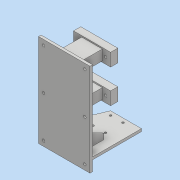
# Autodesk Inventor part: Giá đỡ động cơ
Saved by Autodesk Inventor 2018 (Build 220112000, 112)
## iProperties
Created: 2020-08-22
Part Number: Giá đỡ động cơ
Material: Generic
Document SubType Name: Modeling
Designer: ASUS
Density: 1 g/cm^3
Appearance: Default
Author: ASUS
Autodesk Inventor part; units mm, degrees
ref_plane "YZ Plane" through (0, 0, 0) normal (1, 0, 0) x (0, 1, 0)
ref_plane "XZ Plane" through (0, 0, 0) normal (0, 1, 0) x (-1, 0, 0)
ref_plane "XY Plane" through (0, 0, 0) normal (0, 0, 1) x (1, 0, 0)
sketch "Sketch1" plane through (0, 0, 0) normal (0, 1, 0) x (-1, 0, 0)
  line L0 (0, 0) -> (100, 0)
  line L1 (100, 0) -> (100, -180)
  line L2 (100, -180) -> (0, -180)
  line L3 (0, -180) -> (0, 0)
  dimension "d0" = 100
  dimension "d1" = 180
  constraints: 8 end point, 2 parallel, 1 horizontal, 1 perpendicular
  measures "d0" distance of L1.end L2.end
  measures "d1" distance of L0.end L1.end
extrude "Extrusion1" add sketch "Sketch1" along normal blind 5
sketch "Sketch2" plane through (0, 5, 0) normal (0, 1, 0) x (1, 0, 0)
  line L0 (0, 160) -> (-100, 160)
  line L1 (-100, 160) -> (-100, 155)
  line L2 (-100, 155) -> (0, 155)
  line L3 (0, 155) -> (0, 160)
  line L4 (0, 180) -> (-100, 180) projected
  point P0 (0, 0)
  dimension "d4" = 100
  dimension "d5" = 5
  dimension "d6" = 20
  constraints: 8 end point, 2 parallel, 1 horizontal, 1 perpendicular
  measures "d4" distance of L2.end L1.end
  measures "d5" distance of L1.end L0.end
  measures "d6" distance between parallel lines of L4 L0
extrude "Extrusion2" add sketch "Sketch2" along normal blind 95
sketch "Sketch5" plane through (0, 5, -160) normal (0, 0, -1) x (-1, 0, 0)
  line L0 (28, 87) -> (52, 87)
  line L1 (52, 87) -> (52, 53)
  line L2 (52, 53) -> (28, 53)
  line L3 (28, 53) -> (28, 87)
  line L4 (28, 87) -> (52, 53) construction
  line L5 (52, 87) -> (28, 53) construction
  line L6 (0, 0) -> (0, 95) projected
  line L7 (0, 95) -> (100, 95) projected
  circle A0 centre (28, 87) radius 2
  circle A1 centre (52, 87) radius 2
  circle A2 centre (28, 53) radius 2
  circle A3 centre (52, 53) radius 2
  point P0 (0, -5)
  point P1 (40, 70)
  point P2 (50, 95)
  dimension "d14" = 24
  dimension "d15" = 34
  dimension "d16" = 40
  dimension "d17" = 25
  dimension "d19" = 4
  dimension "d20" = 4
  dimension "d21" = 4
  dimension "d22" = 4
  constraints: 12 end point, 4 centre point, 4 coincident, 2 midpoint, 2 parallel, 1 horizontal, 1 perpendicular
  measures "d14" distance of L1.end L2.end
  measures "d15" distance of L0.end L1.end
  measures "d16" distance from line of L6 point (40, 70)
  measures "d17" distance from line of L7 point (40, 70)
  measures "d19" diameter of A0
  measures "d20" diameter of A1
  measures "d21" diameter of A2
  measures "d22" diameter of A3
extrude "Extrusion4" cut sketch "Sketch5" against normal blind 95 contours L3 A0 L0 | L0 A0 L3 | A1 L1 L0 | L0 L1 A1 | A2 L2 L3 | L3 L2 A2 | A3 L2 L1 | L1 L2 A3
sketch "Sketch12" plane through (0, 5, -160) normal (0, 0, -1) x (-1, 0, 0)
  line L0 (0, 95) -> (100, 95) projected
  line L1 (100, 95) -> (60, 95)
  line L2 (100, 0) -> (0, 0) projected
  line L3 (60, 95) -> (100, 0)
  line L4 (100, 0) -> (100, 95)
  point P0 (0, -5)
  dimension "d72" = 40
  constraints: 6 end point, 1 perpendicular, 1 point on line
  measures "d72" distance of L0.end L1.end
extrude "Extrusion10" cut sketch "Sketch12" against normal blind 14
sketch "Sketch13" plane through (0, 5, 0) normal (0, 1, 0) x (1, 0, 0)
  line L0 (-20, 23) -> (-60, 23)
  line L1 (-60, 23) -> (-60, 3)
  line L2 (-60, 3) -> (-20, 3)
  line L3 (-20, 3) -> (-20, 23)
  line L4 (-20, 23) -> (-60, 3) construction
  line L5 (-60, 23) -> (-20, 3) construction
  line L6 (-100, 0) -> (0, 0) projected
  line L7 (0, 0) -> (0, 155) projected
  line L8 (-20, 88) -> (-60, 88)
  line L9 (-60, 88) -> (-60, 68)
  line L10 (-60, 68) -> (-20, 68)
  line L11 (-20, 68) -> (-20, 88)
  line L12 (-20, 88) -> (-60, 68) construction
  line L13 (-60, 88) -> (-20, 68) construction
  point P0 (-40, 13)
  point P1 (-40, 78)
  dimension "d76" = 40
  dimension "d77" = 20
  dimension "d78" = 3
  dimension "d79" = 40
  dimension "d80" = 40
  dimension "d81" = 20
  dimension "d82" = 45
  dimension "d83" = 40
  constraints: 24 end point, 4 midpoint, 4 parallel, 2 horizontal, 2 perpendicular
  measures "d76" distance of L2.end L1.end
  measures "d77" distance of L1.end L0.end
  measures "d78" distance between parallel lines of L6 L2
  measures "d79" distance from line of L7 point (-40, 13)
  measures "d80" distance of L10.end L9.end
  measures "d81" distance of L9.end L8.end
  measures "d82" distance between parallel lines of L0 L10
  measures "d83" distance from line of L7 point (-40, 78)
extrude "Extrusion11" add sketch "Sketch13" along normal blind 39
sketch "Sketch14" plane through (0, 44, 0) normal (0, 1, 0) x (1, 0, 0)
  line L0 (-4, 90.5) -> (-76, 90.5)
  line L1 (-76, 90.5) -> (-76, 65.5)
  line L2 (-76, 65.5) -> (-4, 65.5)
  line L3 (-4, 65.5) -> (-4, 90.5)
  line L4 (-4, 90.5) -> (-76, 65.5) construction
  line L5 (-76, 90.5) -> (-4, 65.5) construction
  line L6 (-20, 88) -> (-60, 88) projected
  line L7 (-20, 68) -> (-20, 88) projected
  line L8 (-4, 25.5) -> (-76, 25.5)
  line L9 (-76, 25.5) -> (-76, 0.5)
  line L10 (-76, 0.5) -> (-4, 0.5)
  line L11 (-4, 0.5) -> (-4, 25.5)
  line L12 (-4, 25.5) -> (-76, 0.5) construction
  line L13 (-76, 25.5) -> (-4, 0.5) construction
  line L14 (-20, 23) -> (-60, 23) projected
  line L15 (-20, 3) -> (-20, 23) projected
  point P0 (0, 0)
  point P1 (-40, 78)
  point P2 (-40, 13)
  dimension "d86" = 72
  dimension "d87" = 25
  dimension "d88" = 10
  dimension "d89" = 20
  dimension "d90" = 72
  dimension "d91" = 25
  dimension "d92" = 10
  dimension "d93" = 20
  constraints: 24 end point, 4 midpoint, 4 parallel, 2 horizontal, 2 perpendicular
  measures "d86" distance of L2.end L1.end
  measures "d87" distance of L1.end L0.end
  measures "d88" distance from line of L6 point (-40, 78)
  measures "d89" distance from line of L7 point (-40, 78)
  measures "d90" distance of L10.end L9.end
  measures "d91" distance of L9.end L8.end
  measures "d92" distance from line of L14 point (-40, 13)
  measures "d93" distance from line of L15 point (-40, 13)
extrude "Extrusion12" add sketch "Sketch14" along normal blind 14
sketch "Sketch16" plane through (0, 5, 0) normal (0, 1, 0) x (1, 0, 0)
  line L0 (0, 180) -> (-100, 180) projected
  line L1 (-38, 160) -> (-43, 160)
  line L2 (-43, 160) -> (-43, 180)
  line L3 (-43, 180) -> (-38, 180)
  line L4 (-38, 180) -> (-38, 160)
  line L5 (0, 160) -> (0, 180) projected
  point P0 (0, 0)
  dimension "d96" = 20
  dimension "d97" = 38
  dimension "d98" = 5
  constraints: 8 end point, 2 parallel, 1 horizontal, 1 perpendicular, 1 point on line
  measures "d96" distance of L3.end L1.start
  measures "d97" distance between parallel lines of L5 L4
  measures "d98" distance between parallel lines of L4 L2
extrude "Extrusion13" add sketch "Sketch16" along normal blind 95
sketch "Sketch18" plane through (0, 5, 0) normal (0, 1, 0) x (1, 0, 0)
  line L0 (-60, 155) -> (-100, 155) projected
  line L1 (-82, 155) -> (-77, 155)
  line L2 (-77, 155) -> (-77, 125)
  line L3 (-77, 125) -> (-82, 125)
  line L4 (-82, 125) -> (-82, 155)
  line L5 (-23, 155) -> (-18, 155)
  line L6 (-18, 155) -> (-18, 125)
  line L7 (-18, 125) -> (-23, 125)
  line L8 (-23, 125) -> (-23, 155)
  line L9 (-100, 155) -> (-100, 0) projected
  line L10 (0, 0) -> (0, 155) projected
  dimension "d103" = 5
  dimension "d104" = 30
  dimension "d105" = 5
  dimension "d106" = 30
  dimension "d107" = 18
  dimension "d108" = 18
  constraints: 16 end point, 4 parallel, 2 horizontal, 2 perpendicular, 2 point on line
  measures "d103" distance of L2.end L3.end
  measures "d104" distance of L1.end L2.end
  measures "d105" distance of L6.end L7.end
  measures "d106" distance of L5.end L6.end
  measures "d107" distance between parallel lines of L9 L4
  measures "d108" distance between parallel lines of L10 L6
extrude "Extrusion15" add sketch "Sketch18" along normal blind 40
sketch "Sketch20" plane through (-43, 5, -180) normal (-1, 0, 0) x (0, 0, 1)
  line L0 (20, 0) -> (20, 95) projected
  line L1 (20, 95) -> (20, 65)
  line L2 (20, 65) -> (15, 65)
  line L3 (0, 0) -> (20, 0) projected
  line L4 (15, 65) -> (0, 0)
  line L5 (0, 95) -> (20, 95) projected
  line L6 (0, 0) -> (0, 95)
  line L7 (0, 95) -> (20, 95)
  point P0 (180, -5)
  dimension "d114" = 30
  dimension "d115" = 5
  constraints: 10 end point, 2 perpendicular, 1 horizontal, 1 point on line
  measures "d114" distance of L0.end L1.end
  measures "d115" distance of L1.end L2.end
extrude "Extrusion17" cut sketch "Sketch20" against normal blind 10 contours L2 L4 L6 L5 L0
sketch "Sketch21" plane through (0, 5, 0) normal (0, 1, 0) x (1, 0, 0)
  circle A0 centre (-90, 10) radius 2.5
  line L0 (-100, 155) -> (-100, 0) projected
  line L1 (-100, 0) -> (0, 0) projected
  circle A1 centre (-10, 10) radius 2.5
  line L2 (0, 0) -> (0, 155) projected
  circle A2 centre (-90, 170) radius 2.5
  line L3 (-43, 180) -> (-100, 180) projected
  line L4 (-100, 180) -> (-100, 160) projected
  circle A3 centre (-10, 170) radius 2.5
  line L5 (0, 180) -> (-38, 180) projected
  line L6 (0, 160) -> (0, 180) projected
  circle A4 centre (-50, 50) radius 2.5
  circle A5 centre (-50, 130) radius 2.5
  dimension "d118" = 5
  dimension "d119" = 10
  dimension "d120" = 10
  dimension "d121" = 5
  dimension "d122" = 10
  dimension "d123" = 10
  dimension "d124" = 5
  dimension "d125" = 10
  dimension "d126" = 10
  dimension "d127" = 5
  dimension "d128" = 10
  dimension "d129" = 10
  dimension "d130" = 5
  dimension "d131" = 5
  dimension "d132" = 50
  dimension "d133" = 50
  constraints: 6 centre point
  measures "d118" diameter of A0
  measures "d119" distance from line of L0 A0.centre
  measures "d120" distance from line of L1 A0.centre
  measures "d121" diameter of A1
  measures "d122" distance from line of L2 A1.centre
  measures "d123" distance from line of L1 A1.centre
  measures "d124" diameter of A2
  measures "d125" distance from line of L3 A2.centre
  measures "d126" distance from line of L4 A2.centre
  measures "d127" diameter of A3
  measures "d128" distance from line of L5 A3.centre
  measures "d129" distance from line of L6 A3.centre
  measures "d130" diameter of A4
  measures "d131" diameter of A5
  measures "d132" distance from line of L1 A4.centre
  measures "d133" distance from line of L3 A5.centre
extrude "Extrusion18" cut sketch "Sketch21" against normal blind 10
sketch "Sketch27" plane through (0, 58, 0) normal (0, 1, 0) x (1, 0, 0)
  circle A0 centre (-66.5, 78) radius 2.5
  line L0 (-4, 90.5) -> (-76, 90.5) projected
  line L1 (-76, 90.5) -> (-76, 65.5) projected
  circle A1 centre (-13.5, 78) radius 2.5
  line L2 (-76, 65.5) -> (-4, 65.5) projected
  circle A2 centre (-66.5, 13) radius 2.5
  line L3 (-76, 25.5) -> (-76, 0.5) projected
  line L4 (-76, 0.5) -> (-4, 0.5) projected
  circle A3 centre (-13.5, 13) radius 2.5
  line L5 (-4, 0.5) -> (-4, 25.5) projected
  point P0 (0, 0)
  dimension "d137" = 5
  dimension "d138" = 12.5
  dimension "d139" = 9.5
  dimension "d140" = 5
  dimension "d141" = 53
  dimension "d142" = 12.5
  dimension "d143" = 5
  dimension "d144" = 9.5
  dimension "d145" = 12.5
  dimension "d146" = 5
  dimension "d147" = 9.5
  dimension "d148" = 12.5
  constraints: 4 centre point
  measures "d137" diameter of A0
  measures "d138" distance from line of L0 A0.centre
  measures "d139" distance from line of L1 A0.centre
  measures "d140" diameter of A1
  measures "d141" distance of A0.centre A1.centre
  measures "d142" distance from line of L2 A1.centre
  measures "d143" diameter of A2
  measures "d144" distance from line of L3 A2.centre
  measures "d145" distance from line of L4 A2.centre
  measures "d146" diameter of A3
  measures "d147" distance from line of L5 A3.centre
  measures "d148" distance from line of L4 A3.centre
extrude "Extrusion19" cut sketch "Sketch27" against normal blind 15
sketch "Sketch28" plane through (-82, 5, -155) normal (-1, 0, 0) x (0, 0, 1)
  line L0 (0, 40) -> (30, 40) projected
  line L1 (30, 40) -> (10, 40)
  line L2 (30, 0) -> (30, 40) projected
  line L3 (10, 40) -> (30, 0)
  line L4 (30, 0) -> (30, 40)
  point P0 (155, -5)
  dimension "d151" = 20
  constraints: 6 end point, 1 collinear, 1 point on line
  measures "d151" distance of L0.end L1.end
extrude "Extrusion20" cut sketch "Sketch28" against normal blind 200
sketch "Sketch29" plane through (0, 0, 0) normal (0, -1, 0) x (1, 0, 0)
  circle A0 centre (-90, -90) radius 2.5
  line L0 (-100, 0) -> (-100, -180) projected
  line L1 (0, 0) -> (-100, 0) projected
  circle A1 centre (-10, -90) radius 2.5
  line L2 (0, -180) -> (0, 0) projected
  dimension "d154" = 5
  dimension "d155" = 10
  dimension "d156" = 90
  dimension "d157" = 5
  dimension "d158" = 10
  dimension "d159" = 90
  constraints: 2 centre point
  measures "d154" diameter of A0
  measures "d155" distance from line of L0 A0.centre
  measures "d156" distance from line of L1 A0.centre
  measures "d157" diameter of A1
  measures "d158" distance from line of L2 A1.centre
  measures "d159" distance from line of L1 A1.centre
extrude "Extrusion21" cut sketch "Sketch29" against normal blind 5
sketch "Sketch30" plane through (0, 0, 0) normal (0, -1, 0) x (1, 0, 0)
  circle A0 centre (-50, -130) radius 2.5 projected
  circle A1 centre (-50, -130) radius 2.5
  circle A2 centre (-50, -50) radius 2.5 projected
  circle A3 centre (-50, -50) radius 2.5
  point P0 (0, 0)
  dimension "d162" = 5
  dimension "d163" = 5
  constraints: 2 centre point, 2 coincident
  measures "d162" diameter of A1
  measures "d163" diameter of A3
extrude "Extrusion22" add sketch "Sketch30" against normal blind 5
body "Solid1"
